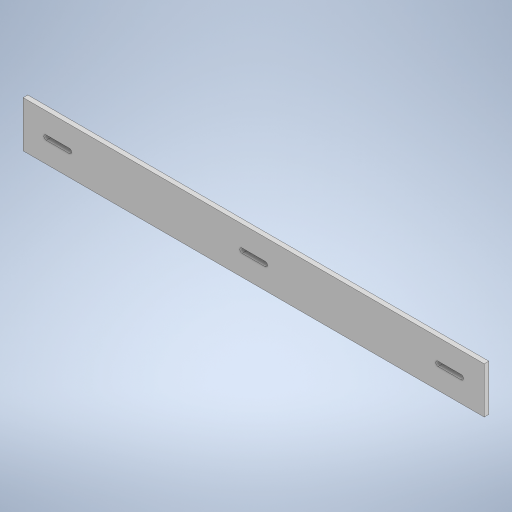
# Autodesk Inventor part: Sides
Saved by Autodesk Inventor 2023 (Build 270158000, 158)
## iProperties
Created: 2022-07-02
Part Number: Sides
Material: Generic
Document SubType Name: Modeling
Designer: Zayed
Density: 1 g/cm^3
Appearance: Default
Author: Zayed
Autodesk Inventor part; units mm, degrees
ref_plane "YZ Plane" through (0, 0, 0) normal (1, 0, 0) x (0, 1, 0)
ref_plane "XZ Plane" through (0, 0, 0) normal (0, 1, 0) x (-1, 0, 0)
ref_plane "XY Plane" through (0, 0, 0) normal (0, 0, 1) x (1, 0, 0)
sketch "Sketch1" plane through (0, 0, 0) normal (0, 0, 1) x (1, 0, 0)
  line L0 (500, 50) -> (-500, 50)
  line L1 (-500, 50) -> (-500, -50)
  line L2 (-500, -50) -> (500, -50)
  line L3 (500, -50) -> (500, 50)
  line L4 (500, 50) -> (-500, -50) construction
  line L5 (-500, 50) -> (500, -50) construction
  point P0 (0, 0)
  dimension "d0" = 1000
  dimension "d1" = 100
  constraints: 12 end point, 2 midpoint, 2 parallel, 1 horizontal, 1 perpendicular
  measures "d0" distance of L2.end L1.end
  measures "d1" distance of L1.end L0.end
sketch "Sketch2" plane through (0, 0, 0) normal (0, 0, 1) x (1, 0, 0)
  line L0 (400, 5) -> (450, 5)
  line L1 (400, -5) -> (450, -5)
  arc A0 (400, 5) -> (400, -5) centre (400, 0) ccw
  arc A1 (450, -5) -> (450, 5) centre (450, 0) ccw
  line L2 (-25, 5) -> (25, 5)
  line L3 (-25, -5) -> (25, -5)
  arc A2 (25, -5) -> (25, 5) centre (25, 0) ccw
  arc A3 (-25, 5) -> (-25, -5) centre (-25, 0) ccw
  line L4 (-450, 5) -> (-400, 5)
  line L5 (-450, -5) -> (-400, -5)
  arc A4 (-400, -5) -> (-400, 5) centre (-400, 0) ccw
  arc A5 (-450, 5) -> (-450, -5) centre (-450, 0) ccw
  point P0 (0, 0)
  constraints: 12 end point, 12 point on circle, 12 tangent, 6 centre point, 2 horizontal
extrude "Extrusion1" add sketch "Sketch1" along normal blind 10
extrude "Extrusion2" cut sketch "Sketch2" along normal blind 10
body "Solid1"
